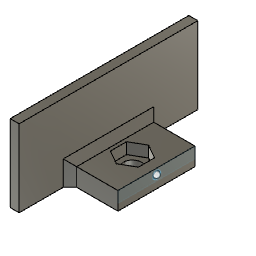
set nut jig (Autodesk Fusion 360 design; units mm, degrees)
Autodesk Fusion 360 part; units mm, degrees
sketch "Sketch1" plane through (0, 0, 0) normal (0, 0, 1) x (1, 0, 0)
  line L0 (5.75, 5.75) -> (-5.75, 5.75) construction
  line L1 (-5.75, 5.75) -> (-5.75, -5.75) construction
  line L2 (-5.75, -5.75) -> (5.75, -5.75) construction
  line L3 (5.75, -5.75) -> (5.75, 5.75) construction
  line L4 (5.75, 5.75) -> (-5.75, -5.75) construction
  line L5 (-5.75, 5.75) -> (5.75, -5.75) construction
  line L6 (5.75, 3.3198) -> (0, 6.6395)
  line L7 (0, 6.6395) -> (-5.75, 3.3198)
  line L8 (-5.75, 3.3198) -> (-5.75, -3.3198)
  line L9 (-5.75, -3.3198) -> (0, -6.6395)
  line L10 (0, -6.6395) -> (5.75, -3.3198)
  line L11 (5.75, -3.3198) -> (5.75, 3.3198)
  circle A0 centre (0, 0) radius 3
  line L12 (-5.75, 5.75) -> (-10.75, 5.75) construction
  line L13 (-10.75, 5.75) -> (-10.75, 17.25)
  line L14 (-10.75, 17.25) -> (-5.75, 17.25)
  line L15 (-5.75, 17.25) -> (-5.75, 5.75) construction
  line L16 (5.75, 5.75) -> (10.75, 5.75) construction
  line L17 (10.75, 5.75) -> (10.75, 17.25)
  line L18 (10.75, 17.25) -> (5.75, 17.25)
  line L19 (5.75, 17.25) -> (5.75, 5.75) construction
  line L20 (-5.75, -5.75) -> (-10.75, -5.75) construction
  line L21 (-10.75, -5.75) -> (-10.75, -17.25)
  line L22 (-10.75, -17.25) -> (-5.75, -17.25)
  line L23 (-5.75, -17.25) -> (-5.75, -5.75) construction
  line L24 (5.75, -5.75) -> (10.75, -5.75) construction
  line L25 (10.75, -5.75) -> (10.75, -17.25)
  line L26 (10.75, -17.25) -> (5.75, -17.25)
  line L27 (5.75, -17.25) -> (5.75, -5.75) construction
  line L28 (-10.75, 17.25) -> (10.75, 17.25)
  line L29 (10.75, 17.25) -> (10.75, -17.25)
  line L30 (10.75, -17.25) -> (-10.75, -17.25)
  line L31 (-10.75, -17.25) -> (-10.75, 17.25)
  line L32 (-6.25, -3.6084) -> (0, -7.2169)
  line L33 (0, -7.2169) -> (6.25, -3.6084)
  line L34 (6.25, -3.6084) -> (6.25, 3.6084)
  line L35 (6.25, 3.6084) -> (0, 7.2169)
  line L36 (0, 7.2169) -> (-6.25, 3.6084)
  line L37 (-6.25, 3.6084) -> (-6.25, -3.6084)
  dimension "d1" = 11.5
  dimension "d2" = 11.5
  dimension "d3" = 6
  dimension "d4" = 5
  dimension "d5" = 11.5
  dimension "d6" = 5
  dimension "d7" = 11.5
  dimension "d8" = 5
  dimension "d9" = 11.5
  dimension "d10" = 5
  dimension "d11" = 11.5
  dimension "d28" = 0.5
  constraint horizontal L0
  constraint perpendicular L0 L1
  constraint parallel L0 L2
  constraint parallel L1 L3
  constraint coincident L4 A0.centre
  constraint coincident L5 A0.centre
  constraint coincident A0.centre origin
  constraint horizontal L12
  constraint vertical L13
  constraint horizontal L14
  constraint vertical L15
  constraint horizontal L16
  constraint vertical L17
  constraint horizontal L18
  constraint vertical L19
  constraint horizontal L20
  constraint vertical L21
  constraint horizontal L22
  constraint vertical L23
  constraint horizontal L24
  constraint vertical L25
  constraint horizontal L26
  constraint vertical L27
  constraint horizontal L28
  constraint vertical L29
  constraint horizontal L30
  constraint vertical L31
  measures "d1" distance of L1.end L2.end
  measures "d2" distance of L0.end L1.end
  measures "d3" diameter of A0
  measures "d4" distance of L0.end L12.end
  measures "d5" distance of L0.end L14.end
  measures "d6" distance of L0.start L16.end
  measures "d7" distance of L0.start L18.end
  measures "d8" distance of L1.end L20.end
  measures "d9" distance of L1.end L22.end
  measures "d10" distance of L2.end L24.end
  measures "d11" distance of L2.end L26.end
extrude "Extrude1" add sketch "Sketch1" along normal blind 5 contours L6 L7 L8 L9 L10 L11 | A0 | L13 L14 L17 L18 L21 L22 L25 L26 L28 L29 L30 L31 | L32 L33 L34 L35 L36 L37 makes body 1
extrude "Extrude6" cut sketch "Sketch1" along normal blind 6 contours L6 L7 L8 L9 L10 L11 | A0 | L32 L33 L34 L35 L36 L37 bodies 1
move_body "Move1" bodies 1 to x (1, 0, 0) y (0, 1, 0) z (0, 0, 1) at (0, 0, -3)
sketch "Sketch2" plane through (10.75, 0, 0) normal (1, 0, 0) x (0, 1, 0)
  line L0 (-17.25, -3) -> (17.25, -3)
  line L1 (17.25, -3) -> (17.25, 2)
  line L2 (17.25, 2) -> (-17.25, 2)
  line L3 (-17.25, 2) -> (-17.25, -3)
  circle A0 centre (0, -0.5) radius 1.5
  dimension "d31" = 3
  measures "d31" diameter of A0
extrude "Extrude8" cut sketch "Sketch2" against normal blind 4.5 contours A0 bodies 1
sketch "Sketch3" plane through (0, 0, -3) normal (0, 0, -1) x (1, 0, 0)
  line L0 (10.75, 17.25) -> (-10.75, 17.25)
  line L1 (-10.75, 17.25) -> (-10.75, -17.25)
  line L2 (-10.75, -17.25) -> (10.75, -17.25)
  line L3 (10.75, -17.25) -> (10.75, 17.25)
  circle A0 centre (0, 0) radius 4
  line L4 (0, -7.2169) -> (-6.25, -3.6084)
  line L5 (-6.25, -3.6084) -> (-6.25, 3.6084)
  line L6 (-6.25, 3.6084) -> (0, 7.2169)
  line L7 (0, 7.2169) -> (6.25, 3.6084)
  line L8 (6.25, 3.6084) -> (6.25, -3.6084)
  line L9 (6.25, -3.6084) -> (0, -7.2169)
  dimension "d18" = 8
  constraint coincident A0.centre origin
  measures "d18" diameter of A0
extrude "Extrude3" add sketch "Sketch3" along normal blind 3 contours L0 L1 L2 L3 | L4 L5 L6 L7 L8 L9 bodies 1
move_body "Move2" bodies 1 to x (1, 0, 0) y (0, 1, 0) z (0, 0, 1) at (0, 0, 1.5)
sketch "Sketch4" plane through (-10.75, 0, 0) normal (-1, 0, 0) x (0, -1, 0)
  line L0 (17.25, -4.5) -> (17.25, 3.5)
  line L1 (17.25, 3.5) -> (-17.25, 3.5)
  line L2 (-17.25, 3.5) -> (-17.25, -4.5)
  line L3 (-17.25, -4.5) -> (17.25, -4.5)
  line L4 (40, 30) -> (-40, 30)
  line L5 (-40, 30) -> (-40, -30)
  line L6 (-40, -30) -> (40, -30)
  line L7 (40, -30) -> (40, 30)
  line L8 (40, 30) -> (-40, -30) construction
  line L9 (-40, 30) -> (40, -30) construction
  dimension "d21" = 80
  dimension "d22" = 60
  constraint horizontal L4
  constraint perpendicular L4 L5
  constraint parallel L4 L6
  constraint parallel L5 L7
  constraint coincident L8 origin
  constraint coincident L9 origin
  measures "d21" distance of L5.end L6.end
  measures "d22" distance of L4.end L5.end
extrude "Extrude4" add sketch "Sketch4" along normal blind 4 contours L0 L1 L2 L3 | L4 L5 L6 L7 bodies 1
extrude "Extrude5" cut 1 faces at (-12.0833, 13.3333, -30) along direction (0, 0, 1) blind 25.5 on bodies 1 bodies 1
chamfer "Chamfer1" distance 3 angle 45 3 edges at (-10.75, 0, 3.5) (-10.75, -17.25, -0.5) (-10.75, 17.25, -0.5) on bodies 1
sketch "Sketch5" plane through (0, 0, 3.5) normal (0, 0, 1) x (-1, 0, 0)
  line L0 (7.75, -17.25) -> (7.75, 17.25)
  line L1 (7.75, 17.25) -> (-10.75, 17.25)
  line L2 (-10.75, 17.25) -> (-10.75, -17.25)
  line L3 (-6.25, 3.6084) -> (0, 7.2169)
  line L4 (0, 7.2169) -> (6.25, 3.6084)
  line L5 (6.25, 3.6084) -> (6.25, -3.6084)
  line L6 (6.25, -3.6084) -> (0, -7.2169)
  line L7 (0, -7.2169) -> (-6.25, -3.6084)
  line L8 (-6.25, -3.6084) -> (-6.25, 3.6084)
  line L9 (-10.75, -17.25) -> (7.75, -17.25)
  line L10 (-10.75, -17.25) -> (-6.25, -17.25)
  line L11 (-6.25, -17.25) -> (-6.25, 17.25)
  line L12 (-6.25, 17.25) -> (-10.75, 17.25)
  line L13 (-10.75, 17.25) -> (-10.75, -17.25)
  constraint horizontal L10
  constraint vertical L11
  constraint horizontal L12
  constraint vertical L13
  constraint coincident L1 L11.end
  constraint coincident L2.end L9.start
extrude "Extrude7" add sketch "Sketch5" against normal blind 7 contours L1 L2 L8 L9 L10 L11 L12 L13 bodies 1
ref_plane "WorkPlane1" through (0, 0, -1.5) normal (0, 0, 1) x (-1, 0, 0)
split "Split1" by plane through (0, 0, -1.5) normal (0, 0, 1) bodies 1 makes body 2 at (-14.75, 13.3333, 9)
sketch "Sketch6" plane through (10.75, 0, 0) normal (1, 0, 0) x (0, 1, 0)
  line L0 (-17.25, -1.5) -> (17.25, -1.5)
  line L1 (17.25, -1.5) -> (17.25, 3.5)
  line L2 (17.25, 3.5) -> (-17.25, 3.5)
  line L3 (-17.25, 3.5) -> (-17.25, -1.5)
  circle A0 centre (0, 1) radius 1.5
  dimension "d37" = 3
  measures "d37" diameter of A0
extrude "Extrude9" cut sketch "Sketch6" against normal blind 4.5 contours A0 bodies 2
combine "Combine1" operation add target body 1 tool bodies 2
